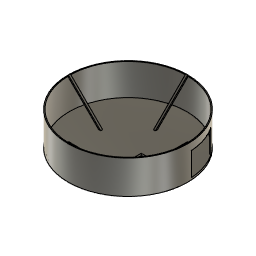
5'SpineMiniFuture v7 (Autodesk Fusion 360 archive; units mm, degrees)
design "BarnTemplate"
Autodesk Fusion 360 part; units mm, degrees
sketch "Sketch1" plane through (0, 0, 0) normal (0, 0, 1) x (1, 0, 0)
  circle A0 centre (0, 0) radius 9144
  line L0 (-9143.9942, 10.2973) -> (-4267.1942, 10.2973) construction
  line L1 (-4114.7942, -142.1027) -> (-4419.5942, -142.1027)
  line L2 (-4419.5942, -142.1027) -> (-4419.5942, 162.6973)
  line L3 (-4419.5942, 162.6973) -> (-4114.7942, 162.6973)
  line L4 (-4114.7942, 162.6973) -> (-4114.7942, -142.1027)
  line L5 (-4114.7942, -142.1027) -> (-4419.5942, 162.6973) construction
  line L6 (-4419.5942, -142.1027) -> (-4114.7942, 162.6973) construction
  line L7 (-162.6973, -4114.7942) -> (142.1027, -4114.7942)
  line L8 (142.1027, -4114.7942) -> (142.1027, -4419.5942)
  line L9 (142.1027, -4419.5942) -> (-162.6973, -4419.5942)
  line L10 (-162.6973, -4419.5942) -> (-162.6973, -4114.7942)
  line L11 (4114.7942, -162.6973) -> (4114.7942, 142.1027)
  line L12 (4114.7942, 142.1027) -> (4419.5942, 142.1027)
  line L13 (4419.5942, 142.1027) -> (4419.5942, -162.6973)
  line L14 (4419.5942, -162.6973) -> (4114.7942, -162.6973)
  line L15 (162.6973, 4114.7942) -> (-142.1027, 4114.7942)
  line L16 (-142.1027, 4114.7942) -> (-142.1027, 4419.5942)
  line L17 (-142.1027, 4419.5942) -> (162.6973, 4419.5942)
  line L18 (162.6973, 4419.5942) -> (162.6973, 4114.7942)
  circle A1 centre (0, 0) radius 9296.4
  point P0 (-4267.1942, 10.2973)
  dimension "d1" = 18288
  dimension "d2" = 4876.8
  dimension "d3" = 304.8
  dimension "d4" = 304.8
  dimension "d6" = 360
  dimension "d7" = 18592.8
  constraint coincident A0.centre A1.centre
  constraint coincident A0 L0.start
  constraint horizontal L0
  constraint horizontal L1
  constraint perpendicular L1 L2
  constraint parallel L1 L3
  constraint parallel L2 L4
  constraint coincident L5 P0
  constraint coincident L6 P0
  constraint coincident P0 L0.end
  constraint concentric A0 A1
  measures "d1" diameter of A0
  measures "d2" distance of L0.start P0
  measures "d3" distance of L2.end L3.end
  measures "d4" distance of L1.end L2.end
  measures "d7" diameter of A1
extrude "Extrude1" add sketch "Sketch1" along normal blind 4876.8 contours A1
extrude "Extrude2" add sketch "Sketch1" against normal blind 304.8 contours A0 | L1 L2 L3 L4 | L7 L8 L9 L10 | L11 L12 L13 L14 | L15 L16 L17 L18 | A1
ref_plane "WorkPlane1" through (9144, 0, 0) normal (1, 0, 0) x (0, 1, 0)
sketch "Sketch2" plane through (9144, 0, 0) normal (1, 0, 0) x (0, 1, 0)
  line L0 (0, 0) -> (0, 4876.8)
  line L1 (-152.4, 4724.4) -> (152.4, 4724.4)
  line L2 (152.4, 4724.4) -> (152.4, 5029.2)
  line L3 (152.4, 5029.2) -> (-152.4, 5029.2)
  line L4 (-152.4, 5029.2) -> (-152.4, 4724.4)
  line L5 (-152.4, 4724.4) -> (152.4, 5029.2) construction
  line L6 (152.4, 4724.4) -> (-152.4, 5029.2) construction
  line L7 (609.6, 0) -> (5181.6, 0)
  line L8 (5181.6, 0) -> (5181.6, 3657.6)
  line L9 (5181.6, 3657.6) -> (609.6, 3657.6)
  line L10 (609.6, 3657.6) -> (609.6, 0)
  point P0 (0, 4876.8)
  dimension "d13" = 4876.8
  dimension "d14" = 304.8
  dimension "d15" = 304.8
  dimension "d18" = 4572
  dimension "d19" = 3657.6
  constraint coincident L0.start origin
  constraint vertical L0
  constraint horizontal L1
  constraint perpendicular L1 L2
  constraint parallel L1 L3
  constraint parallel L2 L4
  constraint coincident L5 P0
  constraint coincident L6 P0
  constraint coincident P0 L0.end
  constraint horizontal L7
  constraint vertical L8
  constraint horizontal L9
  constraint vertical L10
  measures "d13" distance of L0.start P0
  measures "d14" distance of L2.end L3.end
  measures "d15" distance of L1.end L2.end
  measures "d18" distance of L7.start L7.end
  measures "d19" distance of L7.start L9.end
loft "Loft1" add profiles "Sketch2", "Sketch1" section 1 contours L1 L2 L3 L4 section 2 contours L11 L12 L13 L14
pattern_circular "C-Pattern1" count 4 over 360 about axis through (0, 0, 1.75) along (0, 0, 1) of "Loft1"
extrude "Extrude4" cut sketch "Sketch2" against normal blind 5486.4 contours L7 L8 L9 L10
extrude "Extrude5" cut 1 faces at (9144, 965.2, 2438.4) along direction (1, 0, 0) blind 2438.4
sketch "Sketch3" plane through (0, 0, 0) normal (0, 0, 1) x (1, 0, 0)
  line L0 (2075.8003, -924.7952) -> (3904.6003, -924.7952)
  line L1 (3904.6003, -924.7952) -> (3904.6003, -10.3952)
  line L2 (3904.6003, -10.3952) -> (2075.8003, -10.3952)
  line L3 (2075.8003, -10.3952) -> (2075.8003, -924.7952)
  dimension "d26" = 1828.8
  dimension "d27" = 914.4
  constraint horizontal L0
  constraint vertical L1
  constraint horizontal L2
  constraint vertical L3
  measures "d26" distance of L0.start L0.end
  measures "d27" distance of L0.start L2.end
extrude "Extrude6" cut sketch "Sketch3" against normal blind 4572
extrude "Extrude3" [suppressed]
